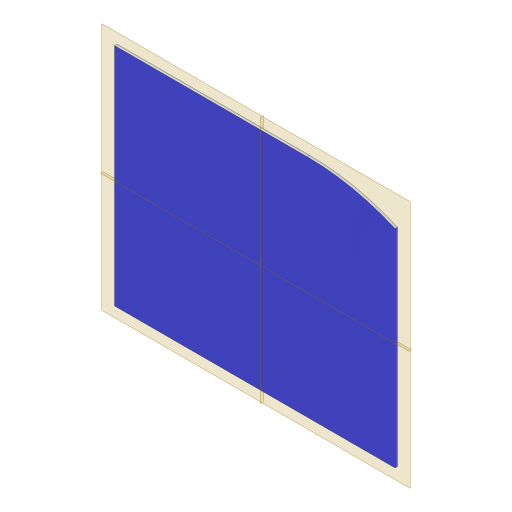
# Autodesk Inventor part: Боковая часть корпуса
Saved by Autodesk Inventor 2023.2 (Build 272271030, 271C)
## iProperties
Created: 2025-04-24
Part Number: Боковая часть корпуса
Material: Типовые
Document SubType Name: Modeling
Designer: Коноваленко
Density: 1 g/cm^3
Appearance: По умолчанию
Author: Коноваленко
Autodesk Inventor part; units mm, degrees
sketch "Эскиз1" plane through (0, 0, 0) normal (0, 0, 1) x (1, 0, 0)
  line L0 (220.2817, 162.8169) -> (220.2817, -177.1831)
  line L1 (220.2817, -177.1831) -> (-239.7183, -177.1831)
  line L2 (-239.7183, -177.1831) -> (-239.7183, 192.8169)
  line L3 (-239.7183, 192.8169) -> (220.2817, -177.1831) construction
  line L4 (220.2817, 162.8169) -> (-239.7183, -177.1831) construction
  line L5 (-332.0278, 0) -> (314.1384, 0) construction
  line L6 (0, 275.7211) -> (0, -252.6671) construction
  line L7 (-239.7183, 192.8169) -> (76.4067, 192.8169)
  arc A0 (220.2817, 162.8169) -> (76.4067, 192.8169) centre (76.4067, -167.1831) ccw
  point P0 (0, 0)
  point P1 (0, 0)
  dimension "d2" = 370
  dimension "d3" = 340
  dimension "d4" = 460
  dimension "d8" = 360
  constraints: 12 end point, 4 point on line, 3 perpendicular, 2 point on circle, 1 centre point, 1 horizontal, 1 tangent
  measures "d2" distance of L1.end L2.end
  measures "d3" distance of L0.start L0.end
  measures "d4" distance of L0.end L1.end
  measures "d8" radius of A0
extrude "Выдавливание1" add sketch "Эскиз1" along normal mid plane 4
